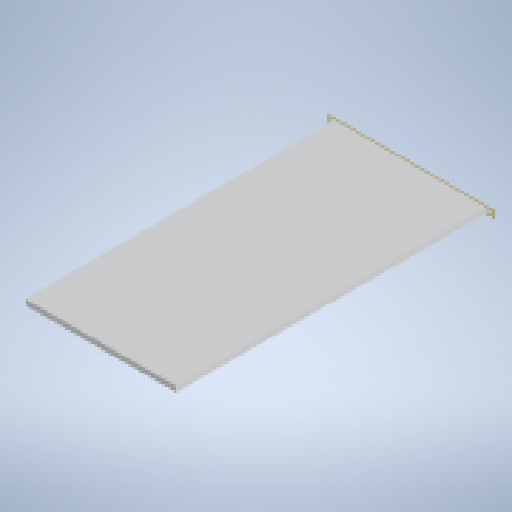
# Autodesk Inventor part: Cover
Saved by Autodesk Inventor 2026 (Build 300175050, 175E)
## iProperties
Created: 2025-07-27
Part Number: Cover
Material: Generic
Document SubType Name: Modeling
Designer: Cupri
Mass: 433.697 g
Surface Area: 1436.71 cm^2
Volume: 433.697 cm^3
Density: 1 g/cm^3
Appearance: Default
Author: Cupri
Autodesk Inventor part; units mm, degrees
ref_plane "YZ Plane" through (0, 0, 0) normal (1, 0, 0) x (0, 1, 0)
ref_plane "XZ Plane" through (0, 0, 0) normal (0, 1, 0) x (-1, 0, 0)
ref_plane "Work Plane1" through (0, 0, 0) normal (0, 0, 1) x (1, 0, 0)
sketch "Sketch1" plane through (0, 0, 0) normal (0, 0, 1) x (1, 0, 0)
  line L0 (-182.3, 6.35) -> (0, 6.35) projected
  line L1 (-182.3, 0) -> (-182.3, 6.35) projected
  line L2 (0, 0) -> (-182.3, 0) projected
  line L3 (0, 0) -> (0, 6.35) projected
ref_plane "Work Plane2" through (-188.6503, -0.0005, 374.65) normal (0, 0, -1) x (0, 1, 0)
extrude "Extrusion1" add sketch "Sketch1" along normal up to surface (374.65 mm away)
body "Solid1"
